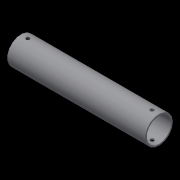
# Autodesk Inventor part: BackPair1PistonShaft
Saved by Autodesk Inventor 2015 SP1 (Build 190203100, 203)
## iProperties
Created: 2014-09-27
Part Number: BackPair1PistonShaft
Material: Generic
Document SubType Name: Modeling
Designer: Inventor
Mass: 2.64222 g
Surface Area: 54.2836 cm^2
Volume: 2.64222 cm^3
Density: 1 g/cm^3
Appearance: Default
Author: Inventor
Autodesk Inventor part; units mm, degrees
ref_plane "YZ Plane" through (0, 0, 0) normal (1, 0, 0) x (0, 1, 0)
ref_plane "XZ Plane" through (0, 0, 0) normal (0, 1, 0) x (-1, 0, 0)
sketch "ShaftProfile" plane through (0, 0, 0) normal (0, 0, 1) x (1, 0, 0)
  line L0 (-56, 0) -> (70, 0) construction
  line L1 (-38, 9) -> (52, 9)
  line L2 (52, 9) -> (52, 0)
  line L3 (-38, 0) -> (-38, 9)
  line L4 (-38, 0) -> (52, 0)
  point P0 (0, 0)
  dimension "d1" = 90
  dimension "d2" = 9
  dimension "d4" = 38
  constraints: 8 end point, 2 horizontal, 2 point on line, 1 parallel, 1 perpendicular
  measures "d1" distance of L1.start L1.end
  measures "d2" distance between parallel lines of L1 L0
  measures "d4" distance from line of L3 point (0, 0)
revolve "ShaftFeature" add sketch "ShaftProfile" angle 360 about axis through (-38, 0, 0) along (1, 0, 0)
sketch "Sketch2" plane through (-38, 0, 0) normal (-1, 0, 0) x (0, 0, 1)
  circle A0 centre (0, 0) radius 9 projected
hole "ShaftHoleFeature" at (-38, 0, 0) direction (1, 0, 0) diameter 16 end through all
ref_plane "MidSidePlane" through (0, 0, 10) normal (0, 0, 1) x (1, 0, 0)
sketch "CapHoles" plane through (0, 0, 10) normal (0, 0, 1) x (1, 0, 0)
  line L0 (52, -9) -> (52, 9) construction
  line L1 (-38, -9) -> (-38, 9) construction
  line L2 (-52, 0) -> (46, 0) construction
  circle A0 centre (-33.5, 0) radius 1.25
  circle A1 centre (47.5, 0) radius 1.25
  dimension "d24" = 2.5
  dimension "d25" = 4.5
  dimension "d26" = 4.5
  constraints: 2 centre point, 2 point on line, 1 equal radius
  measures "d24" diameter of A0
  measures "d25" distance from line of L1 A0.centre
  measures "d26" distance from line of L0 A1.centre
extrude "CapHolesFeature" cut sketch "CapHoles" against normal through all
equation "\"d26\" = d25"
